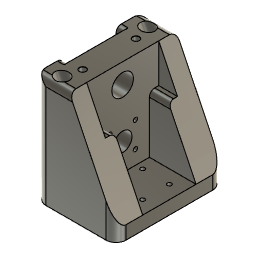
Moving Load Cell Mount Mk2 v23 (Autodesk Fusion 360 design; units mm, degrees)
Autodesk Fusion 360 part; units mm, degrees
note: some values were not read from the file. Chosen so that the rebuilt part matches the saved one: which face or edge a step refers to.
sketch "Sketch1" plane through (0, 0, 0) normal (0, 0, 1) x (1, 0, 0)
  line L0 (0, 0) -> (60, 0)
  line L1 (60, 0) -> (60, 80)
  line L2 (60, 80) -> (0, 80)
  line L3 (0, 80) -> (0, 0)
  dimension "d71" = 80
  dimension "d81" = 60
  constraint horizontal L0
  constraint vertical L1
  constraint horizontal L2
  constraint vertical L3
  constraint coincident L0.start L3.end
  measures "d71" distance of L0 L2
  measures "d81" distance of L1 L3
extrude "Extrude1" add sketch "Sketch1" along normal blind 10
sketch "Sketch2" plane through (0, 0, 10) normal (0, 0, 1) x (-1, 0, 0)
  line L0 (0, -80) -> (0, 0)
  line L1 (0, 0) -> (-60, 0)
  line L2 (-60, 0) -> (-60, -80)
  line L3 (-60, -80) -> (0, -80)
  line L4 (-25, -80) -> (-5, -80)
  line L5 (-5, -80) -> (-5, 0)
  line L6 (-5, 0) -> (-25, 0)
  line L7 (-25, 0) -> (-25, -80)
  dimension "d70" = 5
  dimension "d84" = 20
  constraint horizontal L4
  constraint vertical L5
  constraint horizontal L6
  constraint vertical L7
  constraint coincident L1 L5.end
  constraint collinear L3 L4
  measures "d70" distance of L0 L5
  measures "d84" distance of L5 L7
extrude "Extrude2" add sketch "Sketch2" along normal blind 72 contours L1 L3 L4 L5 L6 L7
sketch "Sketch3" plane through (25, 0, 0) normal (1, 0, 0) x (0, 1, 0)
  line L0 (0, 0) -> (80, 0)
  line L1 (80, 0) -> (80, 10)
  line L2 (80, 82) -> (0, 82)
  line L3 (0, 10) -> (0, 0)
  circle A0 centre (40, 30) radius 7
  circle A1 centre (30.4541, 20.4541) radius 1.6
  circle A2 centre (49.5459, 20.4541) radius 1.6
  circle A3 centre (40, 30) radius 13.5 construction
  line L4 (40, 30) -> (30.4541, 39.5459) construction
  line L5 (40, 30) -> (53.5, 30) construction
  line L6 (40, 30) -> (49.5459, 39.5459) construction
  line L7 (40, 30) -> (53.5, 30) construction
  line L8 (40, 30) -> (30.4541, 20.4541) construction
  line L9 (40, 30) -> (49.5459, 20.4541) construction
  circle A4 centre (30.4541, 39.5459) radius 1.6
  circle A5 centre (49.5459, 39.5459) radius 1.6
  line L10 (80, 10) -> (0, 10)
  line L11 (0, 10) -> (80, 10)
  line L12 (80, 10) -> (80, 82)
  line L13 (0, 82) -> (0, 10)
  dimension "d5" = 14
  dimension "d6" = 30
  dimension "d7" = 40
  dimension "d9" = 3.2
  dimension "d11" = 3.2
  dimension "d19" = 27
  dimension "d20" = 135
  dimension "d21" = 45
  dimension "d22" = 3.2
  dimension "d23" = 3.2
  constraint concentric A0 A3
  constraint coincident A2.centre A3
  constraint coincident A1.centre A3
  constraint horizontal L5
  constraint coincident A0.centre A3.centre
  constraint horizontal L7
  constraint coincident A3 L4.end
  constraint coincident A3 L6.end
  constraint coincident A3 A1.centre
  constraint parallel L6 L8
  constraint coincident A3 A2.centre
  constraint perpendicular L6 L9
  constraint coincident A1.centre L8.end
  constraint coincident A2.centre L9.end
  constraint coincident L4.end A4.centre
  constraint coincident L6.end A5.centre
  measures "d5" diameter of A0
  measures "d6" distance of L0 A0.centre
  measures "d7" distance of L3 A0.centre
  measures "d9" diameter of A1
  measures "d11" diameter of A2
  measures "d19" diameter of A3
  measures "d20" angle of L4 L5
  measures "d21" angle of L6 L7
  measures "d22" diameter of A4
  measures "d23" diameter of A5
extrude "Extrude3" cut sketch "Sketch3" against normal blind 20 contours A0 | A1 | A2 | A4 | A5
sketch "Sketch4" plane through (5, 0, 0) normal (-1, 0, 0) x (0, -1, 0)
  line L0 (-80, 10) -> (0, 10)
  line L1 (0, 10) -> (0, 82)
  line L2 (0, 82) -> (-80, 82)
  line L3 (-80, 82) -> (-80, 10)
  circle A0 centre (-40, 67) radius 8.1
  line L4 (0, 10) -> (0, 82)
  circle A1 centre (-30.4541, 20.4541) radius 1.6
  circle A2 centre (-49.5459, 20.4541) radius 1.6
  circle A3 centre (-30.4541, 39.5459) radius 1.6
  circle A4 centre (-49.5459, 39.5459) radius 1.6
  circle A5 centre (-40, 30) radius 7
  dimension "d26" = 16.2
  dimension "d69" = 15
  dimension "d72" = 40
  measures "d26" diameter of A0
  measures "d69" distance of L2 A0.centre
  measures "d72" distance of A0.centre L4
extrude "Extrude4" cut sketch "Sketch4" against normal blind 20 contours A0
sketch "Sketch5" plane through (0, 0, 10) normal (0, 0, 1) x (-1, 0, 0)
  line L0 (-5, 0) -> (-5, -80)
  line L1 (-5, -80) -> (0, -80)
  line L2 (0, -80) -> (0, 0)
  line L3 (0, 0) -> (-5, 0)
  circle A0 centre (-30, -50) radius 1.6
  circle A1 centre (-50, -50) radius 1.6
  circle A2 centre (-30, -30) radius 1.6
  circle A3 centre (-50, -30) radius 1.6
  dimension "d30" = 3.2
  dimension "d31" = 3.2
  dimension "d32" = 3.2
  dimension "d33" = 3.2
  dimension "d34" = 30
  dimension "d35" = 20
  dimension "d36" = 30
  dimension "d37" = 20
  dimension "d41" = 30
  dimension "d42" = 30
  dimension "d43" = 30
  dimension "d130" = 20
  measures "d30" diameter of A0
  measures "d31" diameter of A1
  measures "d32" diameter of A2
  measures "d33" diameter of A3
  measures "d34" distance of L2 A0.centre
  measures "d35" distance of A0.centre A1.centre
  measures "d36" distance of L2 A2.centre
  measures "d37" distance of A2.centre A3.centre
  measures "d41" distance of L1 A1.centre
  measures "d42" distance of L3 A3.centre
  measures "d43" distance of L1 A0.centre
  measures "d130" distance of A0.centre A2.centre
extrude "Extrude5" cut sketch "Sketch5" against normal blind 10 contours A0 | A1 | A2 | A3
sketch "Sketch7" plane through (0, 0, 10) normal (0, 0, 1) x (-1, 0, 0)
  line L0 (-5, 0) -> (-5, -80)
  line L1 (-5, -80) -> (0, -80)
  line L2 (0, -80) -> (0, 0)
  line L3 (0, 0) -> (-5, 0)
  line L4 (0, -80) -> (-60, -80)
  line L5 (-60, -80) -> (-60, -60)
  line L6 (-60, -60) -> (0, -60)
  line L7 (0, -60) -> (0, -80)
  line L8 (-60, 0) -> (-60, -80)
  line L9 (0, 0) -> (-60, 0)
  line L10 (-60, 0) -> (-60, -20)
  line L11 (-60, -20) -> (0, -20)
  line L12 (0, -20) -> (0, 0)
  dimension "d50" = 20
  dimension "d73" = 20
  constraint horizontal L4
  constraint vertical L5
  constraint horizontal L6
  constraint vertical L7
  constraint coincident L1.end L2.start
  constraint collinear L5 L8
  constraint horizontal L9
  constraint vertical L10
  constraint horizontal L11
  constraint vertical L12
  constraint coincident L8 L10.end
  constraint coincident L2.end L3.start
  measures "d50" distance of L1.end L6.end
  measures "d73" distance of L9 L11
extrude "Extrude7" add sketch "Sketch7" along normal blind 72 contours L0 L2 L3 L9 L11 L12 | L0 L8 L9 L10 L11 | L0 L1 L2 L4 L6 L7 | L0 L4 L5 L6 L8
chamfer "Chamfer1" distance 35 distance2 72 2 edges at (60, 70, 82) (60, 10, 82) measured on face at (28.3333, 73.3333, 82) measured on face at (28.3333, 73.3333, 82)
fillet "Fillet1" radius 7.5 4 edges at (0, 0, 41) (0, 80, 41) (60, 0, 5) (60, 80, 5)
sketch "Sketch8" plane through (0, 0, 0) normal (-1, 0, 0) x (0, -1, 0)
  line L0 (-72.5, 82) -> (-72.5, 0)
  line L1 (-72.5, 0) -> (-7.5, 0)
  line L2 (-7.5, 0) -> (-7.5, 82)
  line L3 (-20, 10) -> (-60, 10)
  circle A0 centre (-50, 6) radius 1.55
  circle A1 centre (-30, 6) radius 1.55
  line L4 (-7.5, 82) -> (-20, 82)
  line L5 (-20, 82) -> (-20, 10)
  line L6 (-60, 10) -> (-60, 82)
  line L7 (-60, 82) -> (-72.5, 82)
  line L8 (-80, 82) -> (-80, 0)
  dimension "d56" = 3.1
  dimension "d57" = 3.1
  dimension "d58" = 20
  dimension "d80" = 30
  measures "d56" diameter of A0
  measures "d57" diameter of A1
  measures "d58" distance of A0.centre A1.centre
  measures "d80" distance of A0.centre L8
extrude "Extrude8" cut sketch "Sketch8" against normal blind 6 contours A0 | A1
sketch "Sketch9" plane through (0, 0, 0) normal (-1, 0, 0) x (0, -1, 0)
  circle A0 centre (-30, 6) radius 1.55
  circle A1 centre (-50, 6) radius 1.55
  line L0 (-72.5, 82) -> (-72.5, 0)
  line L1 (-72.5, 0) -> (-7.5, 0)
  line L2 (-7.5, 0) -> (-7.5, 82)
  line L3 (-20, 10) -> (-60, 10)
  circle A2 centre (-50, 6) radius 3
  circle A3 centre (-30, 6) radius 3
  line L4 (-53, 6) -> (-47, 6)
  line L5 (-47, 6) -> (-47, 0)
  line L6 (-47, 0) -> (-53, 0)
  line L7 (-53, 0) -> (-53, 6)
  line L8 (-33, 6) -> (-27, 6)
  line L9 (-27, 6) -> (-27, 0)
  line L10 (-27, 0) -> (-33, 0)
  line L11 (-33, 0) -> (-33, 6)
  line L12 (-7.5, 82) -> (-20, 82)
  line L13 (-20, 82) -> (-20, 10)
  line L14 (-60, 10) -> (-60, 82)
  line L15 (-60, 82) -> (-72.5, 82)
  dimension "d82" = 6
  dimension "d83" = 6
  constraint concentric A1 A2
  constraint concentric A0 A3
  constraint horizontal L4
  constraint vertical L5
  constraint horizontal L6
  constraint vertical L7
  constraint coincident L1 L5.end
  constraint coincident A2 L4.start
  constraint horizontal L8
  constraint vertical L9
  constraint horizontal L10
  constraint vertical L11
  constraint coincident L1 L9.end
  constraint coincident A3 L8.start
  constraint tangent A2 L5
  constraint tangent A3 L9
  constraint tangent A2 L7
  constraint tangent A3 L11
  measures "d82" diameter of A2
  measures "d83" diameter of A3
extrude "Extrude9" add sketch "Sketch9" along normal blind 2 contours A0 A3 L8 | A0 A3 L8 | L1 A3 L9 L10 L11 | L1 A2 L5 L6 L7 | A1 A2 L4 | A1 A2 L4
ref_plane "WorkPlane1" through (5, 30, 6) normal (-1, 0, 0) x (0, -1, 0)
sketch "Sketch10" plane through (5, 20, 6) normal (-1, 0, 0) x (0, 1, 0)
  circle A0 centre (30, 0) radius 1.55
  circle A1 centre (10, 0) radius 1.55
  line L0 (27.15, -1.6454) -> (30, -3.2909)
  line L1 (30, -3.2909) -> (32.85, -1.6454)
  line L2 (32.85, -1.6454) -> (32.85, 1.6454)
  line L3 (32.85, 1.6454) -> (30, 3.2909)
  line L4 (30, 3.2909) -> (27.15, 1.6454)
  line L5 (27.15, 1.6454) -> (27.15, -1.6454)
  line L6 (32.85, -1.6454) -> (27.15, -1.6454)
  line L7 (27.15, -1.6454) -> (27.15, -4.0523)
  line L8 (27.15, -4.0523) -> (32.85, -4.0523)
  line L9 (32.85, -4.0523) -> (32.85, -1.6454)
  line L10 (12.85, 1.6454) -> (10, 3.2909)
  line L11 (10, 3.2909) -> (7.15, 1.6454)
  line L12 (7.15, 1.6454) -> (7.15, -1.6454)
  line L13 (7.15, -1.6454) -> (10, -3.2909)
  line L14 (10, -3.2909) -> (12.85, -1.6454)
  line L15 (12.85, -1.6454) -> (12.85, 1.6454)
  line L16 (12.85, -1.6454) -> (7.15, -1.6454)
  line L17 (7.15, -1.6454) -> (7.15, -4.2829)
  line L18 (7.15, -4.2829) -> (12.85, -4.2829)
  line L19 (12.85, -4.2829) -> (12.85, -1.6454)
  point P0 (30, 0)
  point P1 (10, 0)
  dimension "d64" = 2.85
  dimension "d65" = 2.85
  constraint coincident P0 A0.centre
  constraint horizontal L6
  constraint vertical L7
  constraint horizontal L8
  constraint vertical L9
  constraint coincident P1 A1.centre
  constraint horizontal L16
  constraint vertical L17
  constraint horizontal L18
  constraint vertical L19
  constraint collinear L12 L17
  constraint collinear L5 L7
  measures "d64" distance of P0 L5
  measures "d65" distance of P1 L15
extrude "Extrude10" cut sketch "Sketch10" along normal blind 2.6 contours A0 | A1 | L0 L1 L6 | L2 L3 L4 L5 L6 | L0 L1 L7 L8 L9 | L10 L11 L12 L15 L16 | L13 L14 L17 L18 L19 | L13 L14 L16
fillet "Fillet2" radius 5 2 edges at (12.5, 80, 82) (12.5, 0, 82)
sketch "Sketch11" plane through (25, 0, 0) normal (1, 0, 0) x (0, 1, 0)
  circle A0 centre (30.4541, 20.4541) radius 1.6
  circle A1 centre (49.5459, 20.4541) radius 1.6
  circle A2 centre (30.4541, 39.5459) radius 1.6
  circle A3 centre (49.5459, 39.5459) radius 1.6
  circle A4 centre (40, 30) radius 7
  line L0 (20, 82) -> (20, 10)
  line L1 (20, 10) -> (60, 10)
  line L2 (60, 10) -> (60, 82)
  line L3 (13, 82) -> (67, 82)
  line L4 (67, 82) -> (67, 53)
  line L5 (67, 53) -> (13, 53)
  line L6 (13, 53) -> (13, 82)
  line L7 (0, 77) -> (0, 25.4286)
  line L8 (60, 82) -> (20, 82)
  circle A5 centre (40, 67) radius 8.1
  dimension "d74" = 29
  dimension "d75" = 54
  dimension "d76" = 13
  constraint horizontal L3
  constraint vertical L4
  constraint horizontal L5
  constraint vertical L6
  measures "d74" distance of L3.start L5.end
  measures "d75" distance of L4 L6
  measures "d76" distance of L6 L7
extrude "Extrude11" cut sketch "Sketch11" along normal blind 35 contours L0 L3 L5 L6 | L2 L3 L4 L5
fillet "Fillet3" radius 4 6 edges at (2.5, 20, 82) (2.5, 60, 82) (2.5, 20, 10) (2.5, 60, 10) (32.0486, 60, 53) (32.0486, 20, 53)
ref_plane "WorkPlane3" through (25, 67, 82) normal (0.437193, 0, -0.899368) x (0, 1, 0)
sketch "Sketch15" plane through (25, 67, 82) normal (0.437193, 0, -0.899368) x (0, 1, 0)
  circle A0 centre (5, -12) radius 2.4
  circle A1 centre (-59, -12) radius 2.4
  line L0 (-54, 0) -> (-62, 0)
  line L1 (8, 0) -> (0, 0)
  line L2 (13, 0) -> (13, -17.9249)
  line L3 (-67, -17.9249) -> (-67, 0)
  dimension "d112" = 4.8
  dimension "d113" = 4.8
  dimension "d114" = 12
  dimension "d115" = 12
  dimension "d116" = 8
  dimension "d117" = 8
  measures "d112" diameter of A0
  measures "d113" diameter of A1
  measures "d114" distance of A1.centre L0
  measures "d115" distance of A0.centre L1
  measures "d116" distance of A0.centre L2
  measures "d117" distance of A1.centre L3
extrude "Extrude14" cut sketch "Sketch15" along normal blind 90 and the other way blind 15
sketch "Sketch16" plane through (25, 67, 82) normal (0.437193, 0, -0.899368) x (0, 1, 0)
  circle A0 centre (5, -12) radius 2.4
  circle A1 centre (-59, -12) radius 2.4
  circle A2 centre (-59, -12) radius 5
  circle A3 centre (5, -12) radius 5
  dimension "d120" = 10
  dimension "d121" = 10
  constraint concentric A1 A2
  constraint concentric A0 A3
  measures "d120" diameter of A2
  measures "d121" diameter of A3
extrude "Extrude16" cut sketch "Sketch16" against normal blind 9
sketch "Sketch17" plane through (0, 0, 82) normal (0, 0, 1) x (-1, 0, 0)
  ellipse E0 centre (-11.6573, -72) end of major axis (-6.0978, -72) minor radius 5 (-7.2097, -75) -> (-16.1049, -75) ccw
  line L0 (-7.2097, -75) -> (-0.4289, -75)
  arc A0 (-0.4289, -75) -> (0, -72.5) centre (-7.5, -72.5) ccw
  line L1 (0, -72.5) -> (0, -64)
  line L2 (0, -64) -> (-5, -64)
  line L3 (-5, -64) -> (-5, -16)
  line L4 (-5, -16) -> (0, -16)
  line L5 (0, -16) -> (0, -7.5)
  arc A1 (0, -7.5) -> (-0.4289, -5) centre (-7.5, -7.5) ccw
  line L6 (-0.4289, -5) -> (-7.2097, -5)
  ellipse E1 centre (-11.6573, -8) end of major axis (-6.0978, -8) minor radius 5 (-16.1049, -5) -> (-7.2097, -5) ccw
  line L7 (-16.1049, -5) -> (-25, -5)
  line L8 (-25, -5) -> (-25, -13)
  line L9 (-25, -13) -> (-25, -67)
  line L10 (-25, -67) -> (-25, -75)
  line L11 (-25, -75) -> (-16.1049, -75)
  circle A2 centre (-15, -60) radius 2.4
  circle A3 centre (-15, -20) radius 2.4
  dimension "d124" = 4.8
  dimension "d125" = 4.8
  dimension "d128" = 10
  dimension "d129" = 10
  measures "d124" diameter of A2
  measures "d125" diameter of A3
  measures "d128" distance of L3 A3.centre
  measures "d129" distance of L3 A2.centre
extrude "Extrude17" cut sketch "Sketch17" against normal blind 82 contours A2 | A3
chamfer "Chamfer2" distance 0.15 angle 45 4 edges at (14.9881, 69.7624, 77.1331) (14.9881, 5.7624, 77.1331) (17.2376, 19.1321, 82) (17.2376, 59.1321, 82)
